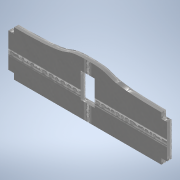
# Autodesk Inventor part: sholder
Saved by Autodesk Inventor 2020.3 (Build 243373000, 373)
## iProperties
Created: 2020-08-06
Part Number: sholder
Material: Generic
Document SubType Name: Modeling
Designer: aditk
Density: 1 g/cm^3
Appearance: Zinc
Author: aditk
Autodesk Inventor part; units mm, degrees
ref_plane "YZ Plane" through (0, 0, 0) normal (1, 0, 0) x (0, 1, 0)
ref_plane "XZ Plane" through (0, 0, 0) normal (0, 1, 0) x (-1, 0, 0)
ref_plane "XY Plane" through (0, 0, 0) normal (0, 0, 1) x (1, 0, 0)
sketch "Sketch1" plane through (0, 0, 0) normal (0, 0, 1) x (1, 0, 0)
  line L0 (-65, -20) -> (65, -20)
  line L1 (70, -15) -> (70, 15)
  line L2 (65, 20) -> (-65, 20)
  line L3 (-70, 15) -> (-70, -15)
  line L4 (65, 20) -> (65, 15)
  line L5 (65, 15) -> (70, 15)
  line L6 (0, 20) -> (0, -20)
  line L7 (65, -20) -> (65, -15)
  line L8 (65, -15) -> (70, -15)
  line L9 (-65, 20) -> (-65, 15)
  line L10 (-65, 15) -> (-70, 15)
  line L11 (-65, -20) -> (-65, -15)
  line L12 (-65, -15) -> (-70, -15)
  point P0 (0, 0)
  constraints: 26 end point, 6 symmetric about line, 2 midpoint, 2 parallel, 2 perpendicular, 1 horizontal, 1 vertical
extrude "Extrusion1" add sketch "Sketch1" along normal blind 4
sketch "Sketch2" plane through (0, 0, 0) normal (0, 0, -1) x (-1, 0, 0)
  arc A0 (-0.55, 20.0026) -> (0.55, 20.0026) centre (0, 19.05) ccw
  line L0 (-0.55, 21.2) -> (-5.25, 21.2)
  line L1 (5.25, 21.2) -> (0.55, 21.2)
  line L2 (6.1, 15.55) -> (6.1, 20.35)
  line L3 (0.55, -10.9) -> (5.25, -10.9)
  line L4 (-5.25, -10.9) -> (-0.55, -10.9)
  arc A1 (0.55, -9.7026) -> (-0.55, -9.7026) centre (0, -8.75) ccw
  line L5 (0.55, -10.9) -> (0.55, -9.7026)
  line L6 (-0.55, -9.7026) -> (-0.55, -10.9)
  line L7 (-6.1, -5.25) -> (-6.1, -10.05)
  line L8 (-6.1, 20.35) -> (-6.1, 15.55)
  arc A2 (-5.25, 21.2) -> (-6.1, 20.35) centre (-5.25, 20.35) ccw
  line L9 (-0.55, 21.2) -> (-0.55, 20.0026)
  line L10 (0.55, 20.0026) -> (0.55, 21.2)
  arc A3 (6.1, 20.35) -> (5.25, 21.2) centre (5.25, 20.35) ccw
  arc A4 (5.25, -10.9) -> (6.1, -10.05) centre (5.25, -10.05) ccw
  line L11 (6.1, -10.05) -> (6.1, -5.25)
  line L12 (6.1, -1.562) -> (6.1, -5.25)
  line L13 (6.1, 15.55) -> (6.1, 1.562)
  circle A5 centre (0, 0) radius 2.25
  line L14 (-6.1, -5.25) -> (-6.1, -1.562)
  line L15 (-6.1, 1.562) -> (-6.1, 15.55)
  line L16 (5.25, 16.4) -> (-5.25, 16.4)
  line L17 (-5.25, -6.1) -> (5.25, -6.1)
  arc A6 (5.25, -6.1) -> (6.1, -5.25) centre (5.25, -5.25) ccw
  arc A7 (-6.1, -5.25) -> (-5.25, -6.1) centre (-5.25, -5.25) ccw
  arc A8 (-6.1, -10.05) -> (-5.25, -10.9) centre (-5.25, -10.05) ccw
  arc A9 (6.1, 15.55) -> (5.25, 16.4) centre (5.25, 15.55) ccw
  arc A10 (-5.25, 16.4) -> (-6.1, 15.55) centre (-5.25, 15.55) ccw
  line L18 (-6.1, 1.562) -> (-6.1, -1.562)
  line L19 (6.1, 1.562) -> (6.1, -1.562)
  circle A11 centre (0, -8.75) radius 1.1
  circle A12 centre (0, 19.05) radius 1.1
  line L20 (-6.1, 15.55) -> (-6.1, 16.4)
  line L21 (-5.25, 16.4) -> (-6.1, 16.4)
  line L22 (5.25, 16.4) -> (6.1, 16.4)
  line L23 (6.1, 15.55) -> (6.1, 16.4)
  line L24 (5.25, -6.1) -> (6.1, -6.1)
  line L25 (-5.25, -6.1) -> (-6.1, -6.1)
  point P0 (-5.25, 21.2)
  point P1 (3.6026, 15)
  point P2 (3.95, 9.45)
  point P3 (0.55, 20.0026)
  point P4 (-0.55, -9.7026)
  point P5 (0.55, -9.7026)
  constraints: 52 end point, 20 point on circle, 13 centre point, 6 point on line, 3 collinear, 3 tangent, 2 coincident, 2 concentric, 1 perpendicular, 1 vertical
sketch "Sketch3" plane through (0, 0, 0) normal (0, 0, -1) x (-1, 0, 0)
  line L0 (-65, 20) -> (65, 20) projected
  line L1 (-65, 20) -> (-20.7877, 20) construction
  line L2 (-20.7877, 20) -> (-20.7877, 27.1367) construction
  line L3 (-20.7877, 27.1367) -> (0, 27.1367) construction
  line L4 (0, 27.1367) -> (20.7877, 27.1367) construction
  line L5 (20.7877, 27.1367) -> (20.7877, 20) construction
  line L6 (20.7877, 20) -> (65, 20) construction
  spline S0 degree 4 poles (-65, 20) (-20.7877, 20) (-20.7877, 27.1367) (0, 27.1367) (20.7877, 27.1367) (20.7877, 20) (65, 20) knots 1 1 1 1 1 2 3 4 4 4 4 4
  line L7 (-65, 15) -> (-65, 20) projected
  line L8 (-65, 20) -> (65, 20)
  point P0 (0, 0)
  constraints: 3 collinear, 2 end point, 3 other
extrude "Extrusion2" add sketch "Sketch3" against normal up to surface (4 mm away)
extrude "Extrusion3" cut sketch "Sketch2" against normal through all contours A12 A0 | L21 A10 L8 | A10 L16 A9 L13 L19 L12 A6 L17 A7 L14 L18 L15 | L2 A9 L22 | A7 L25 L7 | L11 L24 A6 | A1 A11 | A5
body "Solid1"
